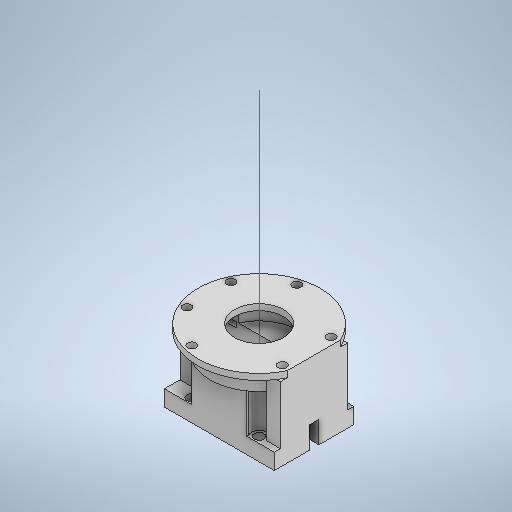
# Autodesk Inventor part: B1
Saved by Autodesk Inventor 2025 (Build 290162000, 162)
## iProperties
Created: 2025-01-02
Part Number: B1
Material: Générique
Document SubType Name: Modeling
Designer: adrie
Density: 1 g/cm^3
Appearance: Par défaut
Author: adrie
Autodesk Inventor part; units mm, degrees
ref_plane "YZ Plane" through (0, 0, 0) normal (1, 0, 0) x (0, 1, 0)
ref_plane "XZ Plane" through (0, 0, 0) normal (0, 1, 0) x (-1, 0, 0)
ref_plane "XY Plane" through (0, 0, 0) normal (0, 0, 1) x (1, 0, 0)
sketch "Esquisse1" plane through (0, 0, 0) normal (0, 1, 0) x (-1, 0, 0)
  circle A0 centre (-27.5, 60) radius 4
  circle A1 centre (27.5, 5) radius 4
  line L0 (-27.5, 60) -> (27.5, 5)
  circle A2 centre (27.5, 60) radius 4
  line L1 (-27.5, 5) -> (27.5, 60)
  line L2 (45, 0) -> (-45, 0)
  line L3 (-45, 0) -> (-45, 65)
  line L4 (-45, 65) -> (45, 65)
  line L5 (45, 65) -> (45, 0)
  line L6 (45, 0) -> (-45, 65) construction
  line L7 (-45, 0) -> (45, 65) construction
  circle A3 centre (0, 32.5) radius 25
  circle A4 centre (-27.5, 5) radius 4
  point P0 (0, 0)
  point P1 (49.3405, -62.4271)
  dimension "d0" = 90
  dimension "d1" = 50
  dimension "d110" = 0
  dimension "d111" = 65
  dimension "d112" = 8
  dimension "d113" = 8
  dimension "d114" = 8
  dimension "d115" = 8
  dimension "d116" = 0
  dimension "d117" = 55
  dimension "d118" = 55
  dimension "d119" = 55
  dimension "d120" = 55
  dimension "d121" = 0
  dimension "d122" = 5
  constraints: 16 end point, 5 centre point, 3 midpoint, 2 coincident, 2 parallel, 1 horizontal, 1 perpendicular
  measures "d0" distance of L3.end L4.end
  measures "d1" diameter of A3
  measures "d110" distance from line of point (0, 0) L2
  measures "d111" distance of L2.end L3.end
  measures "d112" diameter of A0
  measures "d113" diameter of A4
  measures "d114" diameter of A2
  measures "d115" diameter of A1
  measures "d116" horizontal distance of point (0, 0) point (0, 32.5)
  measures "d117" horizontal distance of L1.start L1.end
  measures "d118" horizontal distance of L1.start L1.end
  measures "d119" horizontal distance of L0.start L0.end
  measures "d120" horizontal distance of L0.start L0.end
  measures "d121" distance from line of point (0, 32.5) L0
  measures "d122" distance from line of L4 L0.start
extrude "Extrusion1" add sketch "Esquisse1" along normal blind 5
sketch "Esquisse2" plane through (0, 5, 0) normal (0, 1, 0) x (1, 0, 0)
  circle A0 centre (-27.5, -60) radius 4 projected
  circle A1 centre (-27.5, -60) radius 6
  circle A2 centre (-27.5, -5) radius 4 projected
  circle A3 centre (-27.5, -5) radius 6
  circle A4 centre (27.5, -5) radius 4 projected
  circle A5 centre (27.5, -5) radius 6
  circle A6 centre (27.5, -60) radius 4 projected
  circle A7 centre (27.5, -60) radius 6
  circle A8 centre (0, -32.5) radius 25 projected
  line L0 (22.5, -56.6834) -> (22.5, -65)
  line L1 (-45, -65) -> (45, -65) projected
  line L2 (-22.5, -56.6834) -> (-22.5, -65)
  line L3 (-22.5, -65) -> (22.5, -65)
  line L4 (-22.5, -8.3166) -> (-22.5, 0)
  line L5 (45, 0) -> (-45, 0) projected
  line L6 (22.5, 3.9407) -> (22.5, -8.3166)
  circle A9 centre (0, -32.5) radius 33.0316
  point P0 (0, 0)
  point P1 (-22.5, -63.3166)
  point P2 (22.5, -63.3166)
  point P3 (22.5, -1.6834)
  point P4 (22.5, 0)
  point P5 (-22.5, -1.6834)
  point P6 (-18.7197, 0)
  point P7 (30.8166, 0)
  point P8 (24.1834, 0)
  point P9 (-30.8166, 0)
  point P10 (-24.1834, 0)
  point P11 (-24.1834, -10)
  point P12 (-24.1834, -55)
  point P13 (24.1834, -55)
  point P14 (24.1834, -10)
  dimension "d4" = 12
  dimension "d5" = 12
  dimension "d6" = 12
  dimension "d7" = 12
  dimension "d123" = 45
  dimension "d124" = 22.5
  dimension "d125" = 45
  dimension "d126" = 22.5
  constraints: 10 end point, 9 coincident, 4 point on line, 3 vertical, 1 parallel, 1 perpendicular, 15 other
  measures "d123" distance between parallel lines of L2 L0
  measures "d124" distance from line of A8.centre L0
  measures "d125" distance between parallel lines of L4 L6
  measures "d126" distance from line of A8.centre L6
extrude "Extrusion2" add sketch "Esquisse2" along normal blind 45 contours A1 A9 L1 L2 | A1 A9 A3 L5 A5 A7 L1 | A9 A7 L0 L1 | A3 L4 L5 A9 | L5 L6 A5 A9 picked at (-17.3205, -62.9325) picked at (17.3205, -62.9325) picked at (-17.3205, -2.0675) picked at (17.3205, -2.0675)
sketch "Esquisse3" plane through (0, 5, 0) normal (0, 1, 0) x (1, 0, 0)
  line L0 (0, -44.5) -> (-35.5, -44.5)
  line L1 (-35.5, -44.5) -> (-35.5, -20.5)
  line L2 (-35.5, -20.5) -> (0, -20.5)
  line L3 (0, -20.5) -> (0, -44.5)
  circle A0 centre (0, -32.5) radius 25 projected
  point P0 (0, 0)
  point P1 (-21.9317, -44.5)
  point P2 (-21.9317, -20.5)
  dimension "d11" = 35.5
  dimension "d12" = 24
  dimension "d13" = 12
  dimension "d14" = 12
  dimension "d127" = 0
  constraints: 8 end point, 2 parallel, 1 coincident, 1 horizontal, 1 perpendicular
  measures "d11" distance of L1.end L2.end
  measures "d12" distance of L2.end L0.start
  measures "d13" distance of A0.centre L0.start
  measures "d14" distance of L2.end A0.centre
  measures "d127" distance from line of A0.centre L3
extrude "Extrusion3" cut sketch "Esquisse3" along normal blind 45 and the other way blind 5 contours L0 L1 L2 A0
sketch "Esquisse4" plane through (0, 5, 0) normal (0, 1, 0) x (1, 0, 0)
  line L0 (-35.5, -20.5) -> (-35.5, -44.5) projected
  line L1 (-35.5, -44.5) -> (16.5, -44.5)
  line L2 (16.5, -44.5) -> (16.5, -20.5)
  line L3 (16.5, -20.5) -> (-35.5, -20.5)
  line L4 (-35.5, -20.5) -> (-35.5, -44.5)
  arc A0 (-21.9317, -44.5) -> (-21.9317, -20.5) centre (0, -32.5) ccw projected
  circle A1 centre (0, -32.5) radius 25
  point P0 (0, 0)
  dimension "d19" = 52
  dimension "d128" = 24
  dimension "d129" = 12
  dimension "d130" = 50
  constraints: 8 end point, 2 parallel, 1 centre point, 1 coincident, 1 horizontal, 1 perpendicular
  measures "d19" distance of L2.end L3.end
  measures "d128" distance between parallel lines of L1 L3
  measures "d129" distance from line of L1 A1.centre
  measures "d130" diameter of A1
extrude "Extrusion4" add sketch "Esquisse4" along normal blind 20 and the other way blind 5 contours A0 L1 L2 L3
sketch "Esquisse5" plane through (0, 5, 0) normal (0, 1, 0) x (1, 0, 0)
  line L0 (16.5, -20.5) -> (16.5, -44.5) projected
  line L1 (16.5, -44.5) -> (8.5, -44.5)
  line L2 (8.5, -44.5) -> (8.5, -36.5)
  line L3 (8.5, -36.5) -> (16.5, -36.5)
  line L4 (16.5, -36.5) -> (16.5, -44.5)
  line L5 (16.5, -20.5) -> (8.5, -20.5)
  line L6 (8.5, -20.5) -> (8.5, -28.5)
  line L7 (8.5, -28.5) -> (16.5, -28.5)
  line L8 (16.5, -28.5) -> (16.5, -20.5)
  line L9 (16.5, -36.5) -> (13.5, -36.5)
  line L10 (16.5, -37.5) -> (16.5, -36.5)
  circle A0 centre (13.25, -37.5) radius 2
  circle A1 centre (13.25, -27.5) radius 2
  point P0 (0, 0)
  point P1 (11.5179, -28.5)
  point P2 (14.9821, -28.5)
  point P3 (16.5, -28.5)
  point P4 (14.9821, -36.5)
  point P5 (11.5179, -36.5)
  dimension "d24" = 8
  dimension "d25" = 8
  dimension "d26" = 8
  dimension "d27" = 8
  dimension "d30" = 4
  dimension "d33" = 4
  dimension "d133" = 1
  dimension "d134" = 3.25
  dimension "d135" = 1
  dimension "d136" = 3.25
  constraints: 20 end point, 4 parallel, 3 horizontal, 2 centre point, 2 perpendicular
  measures "d24" distance of L2.end L3.end
  measures "d25" distance of L1.end L2.end
  measures "d26" distance of L5.end L6.end
  measures "d27" distance of L6.end L7.end
  measures "d30" diameter of A0
  measures "d33" diameter of A1
  measures "d133" distance from line of L7 A1.centre
  measures "d134" distance from line of L0 A1.centre
  measures "d135" distance from line of L3 A0.centre
  measures "d136" distance from line of L0 A0.centre
extrude "Extrusion5" add sketch "Esquisse5" along normal blind 20 and the other way blind 5 contours L0 L7 A1 L6 L5 | L0 L1 L2 L3 A0
sketch "Esquisse6" plane through (0, 5, 0) normal (0, 1, 0) x (1, 0, 0)
  circle A0 centre (-33, -15.5) radius 1.5
  circle A1 centre (-33, -49.5) radius 1.5
  line L0 (-30.7748, -44.5) -> (-35.5, -44.5) projected
  line L1 (-35.5, -20.5) -> (-30.7748, -20.5) projected
  line L2 (-35.5, -44.5) -> (-35.5, -20.5) projected
  line L3 (-35.5, -20.5) -> (-35.5, -12.7811)
  line L4 (-35.5, -12.7811) -> (-26.5, -12.7811)
  arc A2 (-24.1834, -10) -> (-30.7748, -20.5) centre (0, -32.5) ccw projected
  line L5 (-35.5, -44.5) -> (-35.5, -52.2189)
  line L6 (-35.5, -52.2189) -> (-26.5, -52.2189)
  arc A3 (-30.7748, -44.5) -> (-24.1834, -55) centre (0, -32.5) ccw projected
  point P0 (-22.2413, -8.1937)
  dimension "d21" = 0
  dimension "d137" = 3
  dimension "d138" = 3
  dimension "d139" = 5
  dimension "d141" = 5
  dimension "d142" = 2.5
  dimension "d143" = 2.5
  dimension "d144" = 9
  dimension "d145" = 9
  constraints: 8 end point, 2 centre point, 2 perpendicular, 2 point on circle, 1 point on line, 1 vertical
  measures "d137" diameter of A1
  measures "d138" diameter of A0
  measures "d139" distance from line of A1.centre L0
  measures "d141" distance from line of L1 A0.centre
  measures "d142" distance from line of A1.centre L2
  measures "d143" distance from line of L2 A0.centre
  measures "d144" distance of L3.end L4.end
  measures "d145" distance of L5.end L6.end
extrude "Extrusion6" add sketch "Esquisse6" along normal blind 28
sketch "Esquisse7" plane through (0, 25, 0) normal (0, 1, 0) x (1, 0, 0)
  line L0 (8.5, -20.5) -> (-35.5, -20.5) projected
  line L1 (-35.5, -20.5) -> (16.5, -20.5)
  line L2 (16.5, -20.5) -> (16.5, -44.5)
  line L3 (16.5, -44.5) -> (-35.5, -44.5)
  line L4 (-35.5, -44.5) -> (-35.5, -20.5)
  arc A0 (-21.9317, -44.5) -> (-21.9317, -20.5) centre (0, -32.5) ccw projected
  circle A1 centre (0, -32.5) radius 25
  point P0 (0, 0)
  dimension "d42" = 52
  dimension "d43" = 24
  dimension "d146" = 50
  constraints: 8 end point, 2 parallel, 1 centre point, 1 coincident, 1 horizontal, 1 perpendicular
  measures "d42" distance of L2.end L3.end
  measures "d43" distance of L1.end L2.end
  measures "d146" diameter of A1
extrude "Extrusion7" add sketch "Esquisse7" along normal blind 25 contours L0 A0 L3 L2 L1
sketch "Esquisse8" plane through (0, 50, 0) normal (0, 1, 0) x (1, 0, 0)
  line L0 (-35.5, -20.5) -> (16.5, -20.5)
  line L1 (16.5, -20.5) -> (16.5, -44.5)
  line L2 (16.5, -44.5) -> (-35.5, -44.5)
  line L3 (-35.5, -44.5) -> (-35.5, -20.5)
  circle A0 centre (0, -32.5) radius 31
  line L4 (-30.7748, -20.5) -> (16.5, -20.5) projected
  line L5 (16.5, -20.5) -> (16.5, -44.5) projected
  arc A1 (24.1834, -55) -> (24.1834, -10) centre (0, -32.5) ccw projected
  point P0 (0, 0)
  point P1 (-28.5832, -44.5)
  point P2 (-28.5832, -20.5)
  dimension "d46" = 52
  dimension "d47" = 24
  dimension "d48" = 62
  dimension "d147" = 0
  dimension "d148" = 0
  dimension "d149" = 0
  dimension "d150" = 0
  constraints: 8 end point, 2 parallel, 1 centre point, 1 horizontal, 1 perpendicular
  measures "d46" distance of L1.end L2.end
  measures "d47" distance of L0.end L1.end
  measures "d48" diameter of A0
  measures "d147" distance between parallel lines of L4 L0
  measures "d148" distance between parallel lines of L5 L1
  measures "d149" distance of A1.centre A0.centre
  measures "d150" distance of A1.centre A0.centre
extrude "Extrusion8" cut sketch "Esquisse8" against normal blind 12.5 contours A0 L2 L1 L0 picked at (21.3333, -32.5)
sketch "Esquisse9" plane through (0, 5, 0) normal (0, 1, 0) x (1, 0, 0)
  circle A0 centre (27.5, -60) radius 4 projected
  circle A1 centre (27.5, -5) radius 4 projected
  line L0 (33.5, -60) -> (45, -60)
  line L1 (-45, -65) -> (45, -65) projected
  line L2 (45, -60) -> (45, -5)
  line L3 (45, -5) -> (33.5, -5)
  arc A2 (-28.5832, -44.5) -> (-28.5832, -20.5) centre (0, -32.5) ccw projected
  line L4 (45, -65) -> (45, 0) projected
  circle A3 centre (0, -32.5) radius 33.0316
  arc A4 (24.1834, -55) -> (22.5, -63.3166) centre (27.5, -60) ccw projected
  circle A5 centre (27.5, -5) radius 6
  circle A6 centre (27.5, -60) radius 6
  point P0 (0, 0)
  point P1 (23.5603, -46.9521)
  point P2 (24.1834, -10)
  dimension "d156" = 12
  dimension "d153" = 0
  dimension "d155" = 12
  constraints: 6 end point, 3 coincident, 2 perpendicular, 1 centre point, 1 horizontal, 1 line through centre, 1 parallel, 5 other
  measures "d153" distance between parallel lines of L4 L2
  measures "d155" diameter of A5
extrude "Extrusion9" add sketch "Esquisse9" along normal blind 32.5 contours A6 A3 A5 L3 L2 L0
sketch "Esquisse10" plane through (0, 37.5, 0) normal (0, 1, 0) x (1, 0, 0)
  circle A0 centre (0, -32.5) radius 31
  arc A1 (-28.5832, -44.5) -> (-28.5832, -20.5) centre (0, -32.5) ccw projected
  circle A2 centre (0, -32.5) radius 40
  line L0 (16.5, -44.5) -> (16.5, -36.5) projected
  line L1 (16.5, -44.5) -> (-38.1576, -44.5)
  line L2 (-38.1576, -44.5) -> (-38.1576, -20.5)
  line L3 (-38.1576, -20.5) -> (16.5, -20.5)
  line L4 (16.5, -20.5) -> (16.5, -44.5)
  line L5 (16.5, -20.5) -> (-28.5832, -20.5) projected
  arc A3 (24.1834, -10) -> (33.5, -5) centre (27.5, -5) ccw projected
  line L6 (45, -60) -> (45, -5) projected
  line L7 (33.5, -5) -> (45, -5)
  line L8 (45, -5) -> (45, -60)
  line L9 (45, -60) -> (33.5, -60)
  arc A4 (33.5, -60) -> (24.1834, -55) centre (27.5, -60) ccw projected
  circle A5 centre (27.5, -5) radius 6
  circle A6 centre (27.5, -60) radius 6
  point P0 (-28.5832, -44.5)
  point P1 (-38.1576, -44.5)
  point P2 (32.1849, -8.7485)
  point P3 (32.1849, -56.2515)
  dimension "d161" = 80
  dimension "d158" = 0
  dimension "d159" = 0
  dimension "d160" = 0
  dimension "d162" = 0
  constraints: 14 end point, 4 coincident, 3 perpendicular, 2 horizontal, 2 horizontal alignment, 2 parallel, 1 centre point, 7 other
  measures "d158" distance of A1.centre A0.centre
  measures "d159" distance of A1.centre A0.centre
  measures "d160" radial gap between concentric circles of A1 A0
  measures "d162" distance between parallel lines of L5 L3
extrude "Extrusion10" add sketch "Esquisse10" along normal blind 15 contours A0 L3 A2 A5 A3 A4 A6 L1 | A2 A3 A5 | A6 A4 A2 | A3 L7 L6 L9 A4 A2 picked at (26.536, -5.8638) picked at (26.536, -59.1361)
sketch "Esquisse11" plane through (0, 52.5, 0) normal (0, 1, 0) x (1, 0, 0)
  circle A0 centre (0, -32.5) radius 31
  circle A1 centre (0, -32.5) radius 40
  arc A2 (-28.5832, -44.5) -> (-28.5832, -20.5) centre (0, -32.5) ccw projected
  line L0 (-28.5832, -20.5) -> (-38.1576, -20.5)
  line L1 (-28.5832, -44.5) -> (-38.1576, -44.5)
  circle A3 centre (0, -32.5) radius 20
  point P0 (0, 0)
  dimension "d165" = 80
  dimension "d187" = 40
  dimension "d197" = 0
  constraints: 4 end point, 3 centre point, 3 coincident, 2 point on circle, 1 horizontal, 1 parallel
  measures "d165" diameter of A1
  measures "d187" diameter of A3
  measures "d197" radial gap between concentric circles of A0 A2
extrude "Extrusion11" add sketch "Esquisse11" along normal blind 5 contours A0 | A0 L0 A1 L1 picked at (-3.5488, -69.1253)
sketch "Esquisse12" plane through (0, 52.5, 0) normal (0, 1, 0) x (1, 0, 0)
  circle A0 centre (0, -32.5) radius 50
  circle A1 centre (0, -32.5) radius 30
  line L0 (45, -65) -> (45, 0) projected
  line L1 (45, -54.2945) -> (45, -10.7055)
  circle A2 centre (0, -32.5) radius 20
  dimension "d167" = 0
  dimension "d168" = 0
  dimension "d169" = 100
  dimension "d170" = 60
  dimension "d188" = 40
  constraints: 3 centre point, 2 coincident, 2 end point, 2 point on circle, 2 point on line
  measures "d167" distance of point (0, -32.5) A0.centre
  measures "d168" distance of point (0, -32.5) A0.centre
  measures "d169" diameter of A0
  measures "d170" diameter of A1
  measures "d188" diameter of A2
extrude "Extrusion12" add sketch "Esquisse12" along normal blind 5 contours L0 A0 picked at (40, -32.5)
sketch "Esquisse13" plane through (0, 5, 0) normal (0, 1, 0) x (1, 0, 0)
  line L0 (-42, 8.1723) -> (-42, -74.6825) construction
  circle A0 centre (-42, -16.7) radius 2.5
  circle A1 centre (-42, -48.3) radius 2.5
  line L1 (-35.5, -44.5) -> (-35.5, -20.5) construction
  line L2 (8.5, -20.5) -> (-35.5, -20.5) construction
  line L3 (-35.5, -44.5) -> (8.5, -44.5) construction
  line L4 (-45, 0) -> (-45, -65) projected
  line L5 (-35.5, -12.7811) -> (-45, -12.7811)
  line L6 (-45, -12.7811) -> (-45, -20.5)
  line L7 (-45, -20.5) -> (-35.5, -20.5)
  line L8 (-35.5, -20.5) -> (-35.5, -12.7811)
  line L9 (-35.5, -44.5) -> (-45, -44.5)
  line L10 (-45, -44.5) -> (-45, -52.2189)
  line L11 (-45, -52.2189) -> (-35.5, -52.2189)
  line L12 (-35.5, -52.2189) -> (-35.5, -44.5)
  point P0 (0, 0)
  dimension "d177" = 5
  dimension "d178" = 5
  dimension "d179" = 6.5
  dimension "d180" = 3.8
  dimension "d183" = 3.8
  dimension "d184" = 7.7189
  dimension "d185" = 7.7189
  constraints: 18 end point, 4 parallel, 4 point on line, 2 centre point, 2 horizontal, 2 perpendicular, 1 vertical
  measures "d177" diameter of A1
  measures "d178" diameter of A0
  measures "d179" distance between parallel lines of L0 L1
  measures "d180" distance from line of A0.centre L2
  measures "d183" distance from line of A1.centre L3
  measures "d184" distance between parallel lines of L7 L5
  measures "d185" distance between parallel lines of L11 L9
extrude "Extrusion13" add sketch "Esquisse13" along normal blind 28
sketch "Esquisse14" plane through (0, 5, 0) normal (0, 1, 0) x (1, 0, 0)
  line L0 (8.5, -44.5) -> (8.5, -36.5) projected
  line L1 (8.5, -28.5) -> (8.5, -20.5) projected
  line L2 (8.5, -36.5) -> (8.5, -28.5)
  line L3 (8.5, -28.5) -> (45, -28.5)
  line L4 (45, -28.5) -> (45, -36.5)
  line L5 (45, -36.5) -> (8.5, -36.5)
  line L6 (16.5, -28.5) -> (16.5, -20.5) projected
  line L7 (16.5, -36.5) -> (16.5, -28.5)
  line L8 (16.5, -28.5) -> (45.1405, -28.5)
  line L9 (45.1405, -28.5) -> (45.1405, -36.5)
  line L10 (45.1405, -36.5) -> (16.5, -36.5)
  line L11 (45, -65) -> (45, 0) projected
  point P0 (0, 0)
  dimension "d186" = 0
  constraints: 16 end point, 6 equal length, 2 perpendicular, 1 point on line
  measures "d186" distance between parallel lines of L4 L11
extrude "Extrusion14" cut sketch "Esquisse14" along normal blind 5 and the other way blind 5 contours L7 L3 L4 L5
sketch "Esquisse15" plane through (0, 57.5, 0) normal (0, 1, 0) x (1, 0, 0)
  line L0 (-12, -103.4809) -> (-12, 37.8934) construction
  circle A0 centre (-12, -75.5) radius 3.5
  circle A1 centre (-12, 10.5) radius 3.5
  point P0 (45.6595, -52.5729)
  point P1 (45.6595, -2.5729)
  point P2 (0, -32.5)
  dimension "d100" = 12
  dimension "d101" = 7
  dimension "d102" = 7
  dimension "d103" = 43
  dimension "d104" = 43
  constraints: 2 centre point, 2 end point, 2 point on line, 1 vertical
  measures "d100" distance from line of point (0, -32.5) L0
  measures "d101" diameter of A0
  measures "d102" diameter of A1
  measures "d103" vertical distance of point (0, -32.5) A0.centre
  measures "d104" vertical distance of A1.centre point (0, -32.5)
extrude "Extrusion15" cut sketch "Esquisse15" against normal blind 10
sketch "Esquisse16" plane through (0, 57.5, 0) normal (0, 1, 0) x (1, 0, 0)
  line L0 (39, 37.1705) -> (39, -124.4417) construction
  circle A0 centre (39, -12.5) radius 3.5
  circle A1 centre (39, -52.5) radius 3.5
  point P0 (0, 0)
  point P1 (0, -32.5)
  dimension "d171" = 39
  dimension "d172" = 7
  dimension "d173" = 7
  dimension "d175" = 20
  dimension "d176" = 20
  constraints: 2 centre point, 2 end point, 2 point on line, 1 vertical
  measures "d171" distance from line of L0 point (0, 0)
  measures "d172" diameter of A1
  measures "d173" diameter of A0
  measures "d175" vertical distance of point (0, -32.5) A0.centre
  measures "d176" vertical distance of A1.centre point (0, -32.5)
extrude "Extrusion16" cut sketch "Esquisse16" against normal blind 35
sketch "Esquisse18" plane through (0, 57.5, 0) normal (0, 1, 0) x (1, 0, 0)
  line L0 (-41, -81.0235) -> (-41, 26.042) construction
  circle A0 centre (-41, -50.5) radius 3.5
  circle A1 centre (-41, -14.5) radius 3.5
  point P0 (0, -32.5)
  dimension "d105" = 7
  dimension "d106" = 7
  dimension "d107" = 18
  dimension "d108" = 18
  dimension "d198" = 41
  constraints: 2 centre point, 2 end point, 2 point on line, 1 vertical
  measures "d105" diameter of A0
  measures "d106" diameter of A1
  measures "d107" vertical distance of point (0, -32.5) A0.centre
  measures "d108" vertical distance of point (0, -32.5) A1.centre
  measures "d198" distance from line of L0 point (0, -32.5)
extrude "Extrusion17" cut sketch "Esquisse18" against normal blind 5
sketch "Sketch19" plane through (0, 0, 0) normal (0, -1, 0) x (1, 0, 0)
  line L0 (-45, 0) -> (-45, 65) projected
  line L1 (-45, 65) -> (45, 65) projected
  line L2 (-45, 0) -> (45, 0)
  line L3 (45, 0) -> (45, 65)
  line L4 (45, 65) -> (-45, 65)
  line L5 (-45, 65) -> (-45, 0)
  line L6 (8.5, 28.5) -> (8.5, 20.5) projected
  line L7 (-35.5, 44.5) -> (8.5, 44.5)
  line L8 (8.5, 44.5) -> (8.5, 20.5)
  line L9 (8.5, 20.5) -> (-35.5, 20.5)
  line L10 (-35.5, 20.5) -> (-35.5, 44.5)
  line L11 (16.5, 36.5) -> (45, 36.5) projected
  line L12 (8.5, 28.5) -> (45, 28.5)
  line L13 (45, 28.5) -> (45, 36.5)
  line L14 (45, 36.5) -> (8.5, 36.5)
  line L15 (8.5, 36.5) -> (8.5, 28.5)
  circle A0 centre (13.25, 37.5) radius 2
  circle A1 centre (13.25, 27.5) radius 2
  arc A2 (14.9821, 36.5) -> (11.5179, 36.5) centre (13.25, 37.5) ccw projected
  arc A3 (11.5179, 28.5) -> (14.9821, 28.5) centre (13.25, 27.5) ccw projected
  circle A4 centre (27.5, 5) radius 4
  circle A5 centre (27.5, 5) radius 4 projected
  circle A6 centre (-27.5, 5) radius 4
  circle A7 centre (-27.5, 5) radius 4 projected
  circle A8 centre (-27.5, 60) radius 4
  circle A9 centre (-27.5, 60) radius 4 projected
  circle A10 centre (27.5, 60) radius 4
  circle A11 centre (27.5, 60) radius 4 projected
  point P0 (0, 0)
  point P1 (8.5, 36.5)
  point P2 (11.5179, 36.5)
  dimension "d189" = 0
  dimension "d190" = 0
  dimension "d191" = 0
  dimension "d192" = 0
  dimension "d193" = 0
  dimension "d194" = 0
  constraints: 24 end point, 6 centre point, 6 parallel, 4 coincident, 4 concentric, 3 horizontal, 3 perpendicular
  measures "d189" distance of A2.centre A0.centre
  measures "d190" distance of A2.centre A0.centre
  measures "d191" radial gap between concentric circles of A2 A0
  measures "d192" distance of A3.centre A1.centre
  measures "d193" distance of A1.centre A3.centre
  measures "d194" radial gap between concentric circles of A1 A3
extrude "Extrusion18" add sketch "Sketch19" along normal blind 8 contours L0 L1 L3 L11 L14 A0 L8 L7 L10 L9 L6 L12 A1 L2
equation "\"d113\" = d112"
equation "\"d114\" = d112"
equation "\"d115\" = d112"
equation "\"d119\" = d117"
equation "\"d135\" = d133"
equation "\"d136\" = d134"
equation "\"d138\" = d137"
equation "\"d178\" = d177"
equation "\"d102\" = d101"
equation "\"d104\" = d103"
equation "\"d173\" = d172"
equation "\"d106\" = d105"
equation "\"d108\" = d107"
